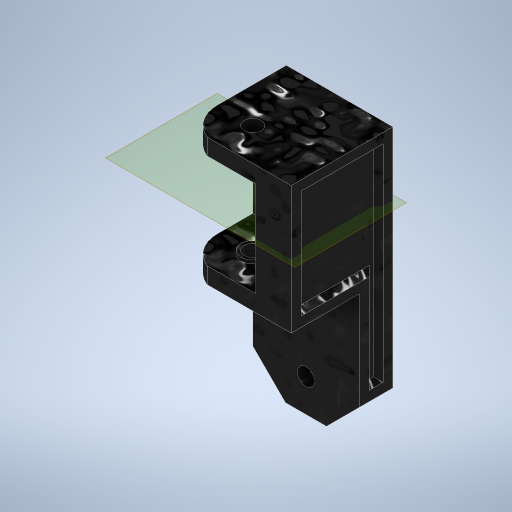
# Autodesk Inventor part: Soporte Poleas Estaticas L
Saved by Autodesk Inventor 2023 (Build 270158000, 158)
## iProperties
Created: 2023-12-10
Part Number: Soporte Poleas Estaticas L
Material: PET Plastic
Document SubType Name: Modeling
Designer: juanp
Density: 1.541 g/cm^3
Appearance: Black
Author: juanp
Autodesk Inventor part; units mm, degrees
ref_plane "YZ Plane" through (0, 0, 0) normal (1, 0, 0) x (0, 1, 0)
ref_plane "XZ Plane" through (0, 0, 0) normal (0, 1, 0) x (-1, 0, 0)
ref_plane "XY Plane" through (0, 0, 0) normal (0, 0, 1) x (1, 0, 0)
sketch "Sketch3" plane through (0, 0, 0) normal (0, 1, 0) x (-1, 0, 0)
  circle A0 centre (0, 0) radius 9.25
  circle A1 centre (0, 0) radius 2.5
  dimension "d6" = 18.5
  dimension "d7" = 5
  constraints: 2 centre point, 2 coincident
  measures "d6" diameter of A0
  measures "d7" diameter of A1
extrude "Extrusion2" add sketch "Sketch3" along normal blind 13
sketch "Sketch4" plane through (0, 13, 0) normal (0, 1, 0) x (1, 0, 0)
  circle A0 centre (0, 0) radius 9.25 projected
  circle A1 centre (0, 0) radius 2.5 projected
  circle A2 centre (0, 0) radius 5
  dimension "d10" = 10
  constraints: 1 centre point, 1 coincident
  measures "d10" diameter of A2
extrude "Extrusion3" add sketch "Sketch4" along normal blind 1 contours A2
sketch "Sketch5" plane through (0, 14, 0) normal (0, 1, 0) x (1, 0, 0)
  circle A0 centre (0, 0) radius 9.25
  circle A1 centre (0, 0) radius 9.25 projected
  circle A2 centre (0, 0) radius 5 projected
  circle A3 centre (0, 0) radius 2.5 projected
  constraints: 1 centre point, 1 coincident, 1 concentric
extrude "Extrusion4" add sketch "Sketch5" along normal blind 13 contours A0 | A2
sketch "Sketch6" plane through (0, 27, 0) normal (0, 1, 0) x (1, 0, 0)
  circle A0 centre (0, 0) radius 9.25 projected
  circle A1 centre (0, 0) radius 2.5 projected
  circle A2 centre (0, 0) radius 5
  dimension "d15" = 10
  constraints: 1 centre point, 1 coincident
  measures "d15" diameter of A2
extrude "Extrusion5" add sketch "Sketch6" along normal blind 1 contours A2
sketch "Sketch7" plane through (0, 0, 0) normal (0, -1, 0) x (1, 0, 0)
  circle A0 centre (0, 0) radius 9.25 projected
  circle A1 centre (0, 0) radius 2.5 projected
  circle A2 centre (0, 0) radius 5
  dimension "d18" = 10
  constraints: 1 centre point, 1 coincident
  measures "d18" diameter of A2
extrude "Extrusion6" add sketch "Sketch7" along normal blind 1 contours A2
sketch "Sketch8" plane through (0, -1, 0) normal (0, -1, 0) x (1, 0, 0)
  line L0 (10, 10) -> (-10, 10) construction
  line L1 (-10, 10) -> (-10, -10) construction
  line L2 (-10, -10) -> (10, -10) construction
  line L3 (10, -10) -> (10, 10) construction
  line L4 (10, 10) -> (-10, -10) construction
  line L5 (-10, 10) -> (10, -10) construction
  line L6 (21.75, 10) -> (-21.75, 10)
  line L7 (-21.75, 10) -> (-21.75, -21)
  line L8 (-21.75, -21) -> (21.75, -21)
  line L9 (21.75, -21) -> (21.75, 10)
  circle A0 centre (0, 0) radius 9.25 construction
  circle A1 centre (0, 0) radius 10.75
  line L10 (-10.75, 0) -> (-10.75, 10)
  line L11 (0, -10.75) -> (21.75, -10.75)
  circle A2 centre (0, 0) radius 2.65
  line L12 (0, -10.75) -> (-21.75, -10.75)
  line L13 (10.75, 10) -> (10.75, -21)
  point P0 (0, 10)
  point P1 (3.9449, 10)
  point P2 (10.75, -10.75)
  point P3 (10.75, 0)
  dimension "d21" = 20
  dimension "d22" = 11
  dimension "d24" = 1.5
  dimension "d25" = 11
  dimension "d26" = 5.3
  constraints: 28 end point, 6 point on line, 5 perpendicular, 4 midpoint, 4 parallel, 3 tangent, 2 centre point, 2 coincident, 2 horizontal, 2 point on circle, 1 vertical
  measures "d21" distance of L2.end L1.end
  measures "d22" distance between parallel lines of L8 L2
  measures "d24" radial gap between concentric circles of A1 A0
  measures "d25" distance between parallel lines of L7 L10
  measures "d26" diameter of A2
extrude "Extrusion7" add sketch "Sketch8" along normal blind 5 separate body contours A1 L6 | L13 L11 A1 | L13 L8 L7 L12 L11 | A1 L10 L6 | L12 L7 L6 L10 A1 picked at (-0.1065, 7.5436)
extrude "Extrusion8" add sketch "Sketch8" along normal blind 45 contours L13 L8 L7 L12 L11 bodies 2
extrude "Extrusion9" add sketch "Sketch8" against normal up to surface (29 mm away) contours L13 L8 L7 L12 L11 | L12 L7 L6 L10 A1 bodies 2
sketch "Sketch9" plane through (-21.75, 28, -21) normal (0, 1, 0) x (1, 0, 0)
  arc A0 (21.75, -10.25) -> (11, -21) centre (21.75, -21) ccw projected
  line L0 (32.5, -10.25) -> (21.75, -10.25) projected
  line L1 (32.5, 0) -> (32.5, -10.25) projected
  line L2 (0, 0) -> (32.5, 0) projected
  line L3 (0, -31) -> (0, 0) projected
  line L4 (11, -31) -> (0, -31) projected
  line L5 (11, -21) -> (11, -31) projected
  circle A1 centre (21.75, -21) radius 2.65 projected
  line L6 (25.6949, -31) -> (11, -31) projected
  line L7 (32.5, -10.25) -> (32.5, -21) projected
  line L8 (11, -21) -> (11, -31) projected
  line L9 (32.5, -10.25) -> (21.75, -10.25) projected
  arc A2 (21.75, -10.25) -> (11, -21) centre (21.75, -21) ccw projected
  arc A3 (25.6949, -31) -> (32.5, -21) centre (21.75, -21) ccw projected
  point P0 (32.5, -10.25)
  point P1 (11, -31)
  point P2 (32.5, -10.25)
  point P3 (11, -31)
extrude "Extrusion10" add sketch "Sketch9" along normal blind 5 bodies 2
sketch "Sketch10" plane through (-21.75, -6, -10.75) normal (0, 0, 1) x (1, 0, 0)
  line L0 (0, 0) -> (32.5, 0) projected
  line L1 (0, 0) -> (0, -40) projected
  line L2 (32.5, -40) -> (0, -40) projected
  line L3 (32.5, 0) -> (32.5, -40) projected
  line L4 (0, 0) -> (32.5, -20) construction
  line L5 (32.5, 39) -> (32.5, -40) projected
  line L6 (32.5, -20) -> (0, -40) construction
  circle A0 centre (16.25, -10) radius 2.65
  circle A1 centre (16.25, -30) radius 2.65
  point P0 (21.75, 6)
  dimension "d35" = 5.3
  dimension "d36" = 5.3
  constraints: 4 end point, 3 midpoint, 2 centre point, 1 point on line
  measures "d35" diameter of A0
  measures "d36" diameter of A1
extrude "Extrusion11" cut sketch "Sketch10" against normal through all contours A0 | A1 bodies 2
chamfer "Chamfer1" distance 10 angle 45 2 edges at (10.75, -46, -15.875) (-21.75, -46, -15.875)
mirror "Mirror1" about plane through (10.75, -1, -21) normal (1, 0, 0) remove original yes bodies 2
sketch "Sketch11" plane through (17.5551, -1, 10) normal (0, 1, 0) x (1, 0, 0)
  circle A0 centre (3.9449, 10) radius 2.65 projected
  circle A1 centre (3.9449, 10) radius 3.65
  point P0 (-17.5551, 10)
  dimension "d42" = 1
  constraints: 1 centre point, 1 coincident
  measures "d42" radial gap between concentric circles of A1 A0
extrude "Extrusion12" add sketch "Sketch11" along normal blind 1 bodies 2
ref_plane "Work Plane1" through (17.5551, 13.5, 10) normal (0, -1, 0) x (1, 0, 0)
mirror "Mirror2" about plane through (17.5551, 13.5, 10) normal (0, -1, 0) of "Extrusion12" bodies 2
sketch "Sketch12" plane through (43.25, 33, -21) normal (0, 0, -1) x (-1, 0, 0)
  line L0 (0, -69) -> (10, -79) projected
  line L1 (10, -79) -> (22.5, -79) projected
  line L2 (22.5, -79) -> (32.5, -69) projected
  line L3 (32.5, 0) -> (32.5, -69) projected
  line L4 (32.5, 0) -> (0, 0) projected
  line L5 (0, 0) -> (0, -69) projected
  circle A0 centre (16.25, -69) radius 2.65 projected
  circle A1 centre (16.25, -49) radius 2.65 projected
  line L6 (3, -67.7574) -> (11.2426, -76)
  line L7 (11.2426, -76) -> (21.2574, -76)
  line L8 (21.2574, -76) -> (29.5, -67.7574)
  line L9 (29.5, -67.7574) -> (29.5, -3)
  line L10 (29.5, -3) -> (3, -3)
  line L11 (3, -3) -> (3, -67.7574)
  circle A2 centre (16.25, -69) radius 5.65
  circle A3 centre (16.25, -49) radius 5.65
  point P0 (43.25, -33)
  dimension "d45" = 3
  dimension "d46" = 3
  dimension "d47" = 3
  constraints: 12 end point, 2 centre point, 5 other
  measures "d45" distance between parallel lines of L5 L11
  measures "d46" radial gap between concentric circles of A0 A2
  measures "d47" radial gap between concentric circles of A1 A3
extrude "Extrusion13" cut sketch "Sketch12" against normal blind 1.5 contours L11 L10 L9 L8 L7 L6 bodies 2
chamfer "Chamfer2" distance 1.5 angle 45 8 edges at (13.75, -2.3787, -19.5) (17.8713, -38.8787, -19.5) (27, -43, -19.5) (32.65, -36, -19.5) (32.65, -16, -19.5) (36.1287, -38.8787, -19.5) (40.25, -2.3787, -19.5) (27, 30, -19.5)
sketch "Sketch13" plane through (43.25, -36, -21) normal (1, 0, 0) x (0, 0, -1)
  line L0 (-10.25, 0) -> (0, 0) projected
  line L1 (0, 69) -> (0, 0) projected
  line L2 (0, 69) -> (-31, 69) projected
  line L3 (-31, 69) -> (-31, 30) projected
  line L4 (-31, 30) -> (-10.25, 30) projected
  line L5 (-10.25, 30) -> (-10.25, 0) projected
  line L6 (-3, 3) -> (-7.25, 3)
  line L7 (-7.25, 3) -> (-7.25, 33)
  line L8 (-7.25, 33) -> (-28, 33)
  line L9 (-28, 33) -> (-28, 66)
  line L10 (-28, 66) -> (-3, 66)
  line L11 (-3, 66) -> (-3, 3)
  point P0 (-21, 36)
  dimension "d53" = 3
  constraints: 12 end point, 5 other
  measures "d53" distance between parallel lines of L1 L11
extrude "Extrusion14" cut sketch "Sketch13" against normal blind 1.5 contours L6 L7 L8 L9 L10 L11 bodies 2
chamfer "Chamfer3" distance 1.5 angle 45 6 edges at (41.75, 30, -5.5) (41.75, -1.5, -18) (41.75, -33, -15.875) (41.75, -18, -13.75) (41.75, 13.5, 7) (41.75, -3, -3.375)
body "Solid2"
body "Solid3"
